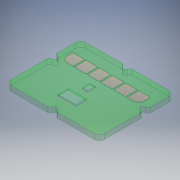
# Autodesk Inventor part: PCB_SMF3300
Saved by Autodesk Inventor 2018 (Build 220112000, 112)
## iProperties
Created: 2020-08-07
Part Number: PCB_SMF3300
Material: Generic
Document SubType Name: Modeling
Designer: sawer
Density: 1 g/cm^3
Appearance: Clear - Green 1
Author: sawer
Autodesk Inventor part; units mm, degrees
ref_plane "YZ Plane" through (0, 0, 0) normal (1, 0, 0) x (0, 1, 0)
ref_plane "XZ Plane" through (0, 0, 0) normal (0, 1, 0) x (-1, 0, 0)
ref_plane "XY Plane" through (0, 0, 0) normal (0, 0, 1) x (1, 0, 0)
sketch "Sketch1" plane through (0, 0, 0) normal (0, 0, 1) x (1, 0, 0)
  line L0 (0, 0) -> (9, 0) construction
  line L1 (9, 0) -> (9, 7.2)
  line L2 (9, 7.2) -> (-9, 7.2)
  line L3 (-9, 7.2) -> (-9, -7.2)
  line L4 (-9, -7.2) -> (9, -7.2)
  line L5 (9, -7.2) -> (9, 0)
  line L6 (9, -7.2) -> (9, 3.05) construction
  dimension "d0" = 9
  dimension "d1" = 7.2
  dimension "d2" = 18
  dimension "d3" = 14.4
  dimension "d4" = 18
  constraints: 14 end point, 3 perpendicular, 1 horizontal, 1 point on line, 1 vertical
  measures "d0" distance of L0.start L0.end
  measures "d1" distance of L0.end L1.end
  measures "d2" distance of L1.end L2.end
  measures "d3" distance of L2.end L3.end
  measures "d4" distance of L3.end L4.end
extrude "Extrusion1" add sketch "Sketch1" along normal blind 1
fillet "Fillet1" radius 1 4 edges at (9, 7.2, 0.5) (9, -7.2, 0.5) (-9, -7.2, 0.5) (-9, 7.2, 0.5)
sketch "Sketch2" plane through (0, 0, 1) normal (0, 0, 1) x (1, 0, 0)
  line L0 (-8, -7.2) -> (8, -7.2) construction
  line L1 (0, -7.2) -> (0, 3.05) construction
  line L2 (0, 3.05) -> (1.27, 3.05) construction
  line L3 (1.27, 3.05) -> (3.81, 3.05) construction
  line L4 (3.81, 3.05) -> (6.35, 3.05) construction
  line L5 (0, 3.05) -> (-1.27, 3.05) construction
  line L6 (-1.27, 3.05) -> (-3.81, 3.05) construction
  line L7 (-3.81, 3.05) -> (-6.35, 3.05) construction
  line L8 (-5.35, 4.2) -> (-7.35, 4.2)
  line L9 (-7.5, 4.05) -> (-7.5, 3.05)
  line L10 (-6.35, 1.9) -> (-5.35, 1.9)
  line L11 (-5.2, 2.05) -> (-5.2, 4.05)
  line L12 (-5.2, 4.2) -> (-7.5, 1.9) construction
  line L13 (-7.5, 4.2) -> (-5.2, 1.9) construction
  line L14 (-2.81, 4.2) -> (-4.81, 4.2)
  line L15 (-4.96, 4.05) -> (-4.96, 1.9)
  line L16 (-4.96, 1.9) -> (-2.81, 1.9)
  line L17 (-2.66, 2.05) -> (-2.66, 4.05)
  line L18 (-2.66, 4.2) -> (-4.96, 1.9) construction
  line L19 (-4.96, 4.2) -> (-2.66, 1.9) construction
  line L20 (-0.27, 4.2) -> (-2.27, 4.2)
  line L21 (-2.42, 4.05) -> (-2.42, 2.05)
  line L22 (-2.27, 1.9) -> (-0.27, 1.9)
  line L23 (-0.12, 2.05) -> (-0.12, 4.05)
  line L24 (-0.12, 4.2) -> (-2.42, 1.9) construction
  line L25 (-2.42, 4.2) -> (-0.12, 1.9) construction
  line L26 (2.27, 4.2) -> (0.27, 4.2)
  line L27 (0.12, 4.05) -> (0.12, 2.05)
  line L28 (0.27, 1.9) -> (2.27, 1.9)
  line L29 (2.42, 2.05) -> (2.42, 4.05)
  line L30 (2.42, 4.2) -> (0.12, 1.9) construction
  line L31 (0.12, 4.2) -> (2.42, 1.9) construction
  line L32 (4.81, 4.2) -> (2.81, 4.2)
  line L33 (2.66, 4.05) -> (2.66, 2.05)
  line L34 (2.81, 1.9) -> (4.81, 1.9)
  line L35 (4.96, 2.05) -> (4.96, 4.05)
  line L36 (4.96, 4.2) -> (2.66, 1.9) construction
  line L37 (2.66, 4.2) -> (4.96, 1.9) construction
  line L38 (7.35, 4.2) -> (5.35, 4.2)
  line L39 (5.2, 4.05) -> (5.2, 2.05)
  line L40 (5.35, 1.9) -> (6.35, 1.9)
  line L41 (7.5, 3.05) -> (7.5, 4.05)
  line L42 (7.5, 4.2) -> (5.2, 1.9) construction
  line L43 (5.2, 4.2) -> (7.5, 1.9) construction
  arc A0 (-7.35, 4.2) -> (-7.5, 4.05) centre (-7.35, 4.05) ccw
  arc A1 (-5.2, 4.05) -> (-5.35, 4.2) centre (-5.35, 4.05) ccw
  arc A2 (-5.35, 1.9) -> (-5.2, 2.05) centre (-5.35, 2.05) ccw
  arc A3 (-4.81, 4.2) -> (-4.96, 4.05) centre (-4.81, 4.05) ccw
  arc A4 (-2.66, 4.05) -> (-2.81, 4.2) centre (-2.81, 4.05) ccw
  arc A5 (-2.81, 1.9) -> (-2.66, 2.05) centre (-2.81, 2.05) ccw
  arc A6 (-2.42, 2.05) -> (-2.27, 1.9) centre (-2.27, 2.05) ccw
  arc A7 (-2.27, 4.2) -> (-2.42, 4.05) centre (-2.27, 4.05) ccw
  arc A8 (-0.27, 1.9) -> (-0.12, 2.05) centre (-0.27, 2.05) ccw
  arc A9 (-0.12, 4.05) -> (-0.27, 4.2) centre (-0.27, 4.05) ccw
  arc A10 (0.27, 4.2) -> (0.12, 4.05) centre (0.27, 4.05) ccw
  arc A11 (0.12, 2.05) -> (0.27, 1.9) centre (0.27, 2.05) ccw
  arc A12 (2.27, 1.9) -> (2.42, 2.05) centre (2.27, 2.05) ccw
  arc A13 (2.42, 4.05) -> (2.27, 4.2) centre (2.27, 4.05) ccw
  arc A14 (2.81, 4.2) -> (2.66, 4.05) centre (2.81, 4.05) ccw
  arc A15 (2.66, 2.05) -> (2.81, 1.9) centre (2.81, 2.05) ccw
  arc A16 (4.81, 1.9) -> (4.96, 2.05) centre (4.81, 2.05) ccw
  arc A17 (4.96, 4.05) -> (4.81, 4.2) centre (4.81, 4.05) ccw
  arc A18 (5.35, 4.2) -> (5.2, 4.05) centre (5.35, 4.05) ccw
  arc A19 (7.5, 4.05) -> (7.35, 4.2) centre (7.35, 4.05) ccw
  arc A20 (5.2, 2.05) -> (5.35, 1.9) centre (5.35, 2.05) ccw
  arc A21 (6.35, 1.9) -> (7.5, 3.05) centre (6.35, 3.05) ccw
  arc A22 (-7.5, 3.05) -> (-6.35, 1.9) centre (-6.35, 3.05) ccw
  point P0 (0, 0)
  dimension "d26" = 10.25
  dimension "d27" = 1.27
  dimension "d28" = 2.54
  dimension "d29" = 2.54
  dimension "d30" = 1.27
  dimension "d31" = 2.54
  dimension "d32" = 2.54
  dimension "d33" = 2.3
  dimension "d34" = 2.3
  dimension "d35" = 2.3
  dimension "d36" = 2.3
  dimension "d37" = 2.3
  dimension "d38" = 2.3
  dimension "d39" = 2.3
  dimension "d40" = 2.3
  dimension "d41" = 2.3
  dimension "d42" = 2.3
  dimension "d43" = 2.3
  dimension "d44" = 2.3
  dimension "d45" = 0.15
  dimension "d48" = 0.15
  dimension "d49" = 1.15
  constraints: 86 end point, 50 point on line, 46 point on circle, 46 tangent, 23 centre point, 20 equal radius, 13 midpoint, 12 parallel, 8 horizontal, 6 perpendicular, 1 vertical
  measures "d26" distance of L1.start L1.end
  measures "d27" distance of L1.end L2.end
  measures "d28" distance of L2.end L3.end
  measures "d29" distance of L3.end L4.end
  measures "d30" distance of L1.end L5.end
  measures "d31" distance of L5.end L6.end
  measures "d32" distance of L6.end L7.end
  measures "d33" distance of L13.end L12.end
  measures "d34" distance of L12.end L13.start
  measures "d35" distance of L19.end L15.end
  measures "d36" distance of L15.end L19.start
  measures "d37" distance of L25.end L24.end
  measures "d38" distance of L24.end L25.start
  measures "d39" distance of L31.end L30.end
  measures "d40" distance of L30.end L31.start
  measures "d41" distance of L37.end L36.end
  measures "d42" distance of L36.end L37.start
  measures "d43" distance of L43.end L42.end
  measures "d44" distance of L42.end L43.start
  measures "d45" radius of A0
  measures "d48" radius of A3
  measures "d49" radius of A21
extrude "Extrusion2" add sketch "Sketch2" along normal blind 0.1
sketch "Sketch3" plane through (0, 0, 1) normal (0, 0, 1) x (1, 0, 0)
  line L0 (-9, 6.2) -> (-9, -6.2) projected
  line L1 (9, -6.2) -> (9, 6.2) projected
  line L2 (8, 7.2) -> (-8, 7.2) projected
  line L3 (0, 7.2) -> (0.5, 7.2)
  line L4 (0.5, 7.2) -> (0.5, 6.825)
  line L5 (0.125, 6.45) -> (-0.125, 6.45)
  line L6 (-0.5, 6.825) -> (-0.5, 7.2)
  line L7 (-8, -7.2) -> (8, -7.2) projected
  line L8 (0, -7.2) -> (-0.5, -7.2)
  line L9 (-0.5, -7.2) -> (-0.5, -6.825)
  line L10 (-0.125, -6.45) -> (0.125, -6.45)
  line L11 (0.5, -6.825) -> (0.5, -7.2)
  line L12 (0.5, -7.2) -> (0, -7.2)
  line L13 (-0.125, 7.2) -> (0, 7.2)
  arc A0 (0.125, 6.45) -> (0.5, 6.825) centre (0.125, 6.825) ccw
  arc A1 (-0.5, 6.825) -> (-0.125, 6.45) centre (-0.125, 6.825) ccw
  arc A2 (0.5, -6.825) -> (0.125, -6.45) centre (0.125, -6.825) ccw
  arc A3 (-0.125, -6.45) -> (-0.5, -6.825) centre (-0.125, -6.825) ccw
  line L14 (0, -6.45) -> (0, -6.132) construction
  line L15 (8, 7.2) -> (9, 7.2) construction
  line L16 (9, 7.2) -> (9, 6.2) construction
  line L17 (9, 7.2) -> (9, 2.2) construction
  line L18 (9, 2.2) -> (8.5, 2.2)
  line L19 (8, 1.7) -> (8, 1.7)
  line L20 (8.5, 1.2) -> (9, 1.2)
  arc A4 (8.5, 2.2) -> (8, 1.7) centre (8.5, 1.7) ccw
  arc A5 (8, 1.7) -> (8.5, 1.2) centre (8.5, 1.7) ccw
  line L21 (-8, 7.2) -> (-9, 7.2) construction
  line L22 (-9, 7.2) -> (-9, 6.2) construction
  line L23 (-9, 7.2) -> (-9, 2.2) construction
  line L24 (-9, 2.2) -> (-8.5, 2.2)
  line L25 (-8, 1.7) -> (-8, 1.7)
  line L26 (-8.5, 1.2) -> (-9, 1.2)
  arc A6 (-8, 1.7) -> (-8.5, 2.2) centre (-8.5, 1.7) ccw
  arc A7 (-8.5, 1.2) -> (-8, 1.7) centre (-8.5, 1.7) ccw
  line L27 (-9, 1.2) -> (-9, 2.2)
  line L28 (9, 1.2) -> (9, 2.2)
  point P0 (0, 0)
  point P1 (0.5, 6.45)
  point P2 (-0.5, 6.45)
  point P3 (-0.5, -6.45)
  point P4 (0.5, -6.45)
  point P5 (8, 2.2)
  point P6 (8, 1.2)
  point P7 (-8, 2.2)
  point P8 (-8, 1.2)
  dimension "d70" = 0.5
  dimension "d71" = 0.75
  dimension "d72" = 1
  dimension "d73" = 0.5
  dimension "d74" = 0.75
  dimension "d75" = 1
  dimension "d76" = 0.75
  dimension "d92" = 5
  dimension "d93" = 1
  dimension "d94" = 1
  dimension "d96" = 5
  dimension "d97" = 1
  dimension "d98" = 1
  constraints: 50 end point, 24 point on line, 17 point on circle, 16 tangent, 11 perpendicular, 8 centre point, 5 equal radius, 4 horizontal, 3 midpoint, 2 vertical, 1 collinear, 1 parallel
  measures "d70" distance of L3.start L3.end
  measures "d71" distance of L3.end point (0.5, 6.45)
  measures "d72" distance of point (0.5, 6.45) point (-0.5, 6.45)
  measures "d73" distance of L8.start L8.end
  measures "d74" distance of L8.end point (-0.5, -6.45)
  measures "d75" distance of point (-0.5, -6.45) point (0.5, -6.45)
  measures "d76" distance of point (0.5, -6.45) L11.end
  measures "d92" distance of L15.end L17.end
  measures "d93" distance of L17.end point (8, 2.2)
  measures "d94" distance of point (8, 2.2) point (8, 1.2)
  measures "d96" distance of L21.end L23.end
  measures "d97" distance of L23.end point (-8, 2.2)
  measures "d98" distance of point (-8, 2.2) point (-8, 1.2)
extrude "Extrusion3" cut sketch "Sketch3" against normal up to surface (1 mm away)
sketch "Sketch5" plane through (0, 0, 1) normal (0, 0, 1) x (1, 0, 0)
  line L0 (-0.125, -6.45) -> (0.125, -6.45) construction
  line L1 (0, -6.45) -> (0, -4.45) construction
  line L2 (0, -4.45) -> (1.75, -4.45)
  line L3 (1.75, -4.45) -> (1.75, -2.45)
  line L4 (1.75, -2.45) -> (-1.75, -2.45)
  line L5 (-1.75, -2.45) -> (-1.75, -4.45)
  line L6 (-1.75, -4.45) -> (0, -4.45)
  line L7 (0, -2.45) -> (0, -0.95) construction
  line L8 (0, -0.95) -> (0.5, -0.95)
  line L9 (0.5, -0.95) -> (0.5, 0.55)
  line L10 (0.5, 0.55) -> (0, 0.55)
  line L11 (0, 0.55) -> (-0.5, 0.55)
  line L12 (-0.5, 0.55) -> (-0.5, -0.95)
  line L13 (-0.5, -0.95) -> (0, -0.95)
  point P0 (0, 0)
  dimension "d78" = 2
  dimension "d80" = 1.75
  dimension "d81" = 2
  dimension "d82" = 3.5
  dimension "d83" = 2
  dimension "d84" = 1.5
  dimension "d85" = 0.5
  dimension "d86" = 1.5
  dimension "d87" = 0.5
  dimension "d88" = 0.5
  constraints: 26 end point, 5 perpendicular, 3 point on line, 3 vertical, 2 midpoint, 1 horizontal
  measures "d78" distance of L1.start L1.end
  measures "d80" distance of L1.end L2.end
  measures "d81" distance of L2.end L3.end
  measures "d82" distance of L3.end L4.end
  measures "d83" distance of L4.end L5.end
  measures "d84" distance of L7.start L7.end
  measures "d85" distance of L7.end L8.end
  measures "d86" distance of L8.end L9.end
  measures "d87" distance of L9.end L10.end
  measures "d88" distance of L10.end L11.end
extrude "Extrusion4" add sketch "Sketch5" along normal blind 0.3
fillet "Fillet4" radius 0.15 4 edges at (0, -0.95, 1.3) (0, 0.55, 1.3) (1.75, -3.45, 1.3) (-1.75, -3.45, 1.3)
fillet "Fillet5" radius 0.5 8 edges at (9, 2.2, 0.5) (0.5, -7.2, 0.5) (-0.5, -7.2, 0.5) (9, 1.2, 0.5) (-9, 2.2, 0.5) (-9, 1.2, 0.5) (0.5, 7.2, 0.5) (-0.5, 7.2, 0.5)
body "Solid1"
